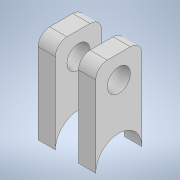
# Autodesk Inventor part: harness attachments
Saved by Autodesk Inventor 2021 (Build 250183000, 183)
## iProperties
Created: 2020-10-11
Part Number: harness attachments
Material: Generic
Document SubType Name: Modeling
Designer: atwaterh
Density: 1 g/cm^3
Appearance: Default
Author: atwaterh
Autodesk Inventor part; units mm, degrees
ref_plane "YZ Plane" through (0, 0, 0) normal (1, 0, 0) x (0, 1, 0)
ref_plane "XZ Plane" through (0, 0, 0) normal (0, 1, 0) x (-1, 0, 0)
ref_plane "XY Plane" through (0, 0, 0) normal (0, 0, 1) x (1, 0, 0)
sketch "Sketch1" plane through (0, 0, 0) normal (1, 0, 0) x (0, 1, 0)
  line L0 (19.05, 12.7) -> (-25.4, 12.7)
  line L1 (-25.4, -12.7) -> (19.05, -12.7)
  line L2 (25.4, -6.35) -> (25.4, 6.35)
  line L3 (25.4, 12.7) -> (-25.4, -12.7) construction
  line L4 (-25.4, 12.7) -> (25.4, -12.7) construction
  circle A0 centre (12.7, 0) radius 6.35
  arc A1 (25.4, 6.35) -> (19.05, 12.7) centre (19.05, 6.35) ccw
  arc A2 (19.05, -12.7) -> (25.4, -6.35) centre (19.05, -6.35) ccw
  arc A3 (-25.4, -12.7) -> (-25.4, 12.7) centre (-25.4, 0) ccw
  point P0 (0, 0)
  dimension "d1" = 25.4
  dimension "d2" = 12.7
  dimension "d3" = 6.35
  dimension "d5" = 12.7
  dimension "d6" = 50.8
  dimension "d7" = 38.1
  constraints: 10 end point, 6 point on circle, 4 centre point, 4 point on line, 4 tangent, 2 midpoint, 1 equal radius, 1 horizontal, 1 parallel, 1 vertical
  measures "d1" distance of L1.start L0.end
  measures "d2" diameter of A0
  measures "d3" radius of A1
  measures "d5" radius of A3
  measures "d6" distance from line of A3.centre L2
  measures "d7" distance of A3.centre A0.centre
extrude "Extrusion1" add sketch "Sketch1" along normal blind 31.75
sketch "Sketch3" plane through (0, -25.4, 12.7) normal (0, 0, 1) x (1, 0, 0)
  line L0 (0, 44.45) -> (0, 0) projected
  line L1 (0, 0) -> (31.75, 0) projected
  line L2 (9.525, 0) -> (22.225, 0)
  line L3 (22.225, 0) -> (22.225, 50.8)
  line L4 (0, 50.8) -> (31.75, 50.8) projected
  line L5 (9.525, 0) -> (9.525, 50.8)
  line L6 (9.525, 50.8) -> (22.225, 50.8)
  point P0 (0, 25.4)
  dimension "d14" = 9.525
  dimension "d15" = 12.7
  constraints: 8 end point, 3 point on line, 2 perpendicular, 1 vertical
  measures "d14" distance of L0.end L2.start
  measures "d15" distance of L2.start L2.end
extrude "Extrusion3" cut sketch "Sketch3" against normal blind 25.4
body "Solid1"
